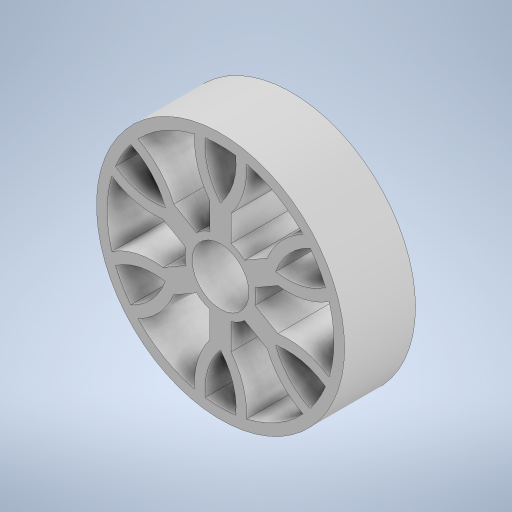
# Autodesk Inventor part: kumandaiç
Saved by Autodesk Inventor 2023 (Build 270158000, 158)
## iProperties
Created: 2023-01-31
Part Number: kumandaiç
Material: Generic
Document SubType Name: Modeling
Designer: Umut Yücesoy
Density: 1 g/cm^3
Appearance: Default
Author: Umut Yücesoy
Autodesk Inventor part; units mm, degrees
ref_plane "YZ Plane" through (0, 0, 0) normal (1, 0, 0) x (0, 1, 0)
ref_plane "XZ Plane" through (0, 0, 0) normal (0, 1, 0) x (-1, 0, 0)
ref_plane "XY Plane" through (0, 0, 0) normal (0, 0, 1) x (1, 0, 0)
sketch "Sketch1" plane through (0, 0, 0) normal (0, 0, 1) x (1, 0, 0)
  circle A0 centre (0, 0) radius 17.5
  circle A1 centre (0, 0) radius 5
  line L0 (0, 5) -> (0, 9)
  arc A2 (0, 9) -> (1.8691, 17.3999) centre (-7.0076, 14.9672) ccw
  arc A3 (1.5, 8.4713) -> (3.471, 17.1523) centre (-7.0076, 14.9672) ccw
  line L1 (1.5, 8.4713) -> (1.5, 4.7697)
  arc A4 (-1.8691, 17.3999) -> (0, 9) centre (7.0076, 14.9672) ccw
  arc A5 (-3.471, 17.1523) -> (-1.5, 8.4713) centre (7.0076, 14.9672) ccw
  line L2 (-1.5, 8.4713) -> (-1.5, 4.7697)
  arc A6 (-6.5864, 5.5347) -> (-13.1189, 11.5821) centre (-16.4658, 1.4148) ccw
  arc A7 (-7.7942, 4.5) -> (-14.1342, 10.3186) centre (-16.4658, 1.4148) ccw
  line L3 (-6.5864, 5.5347) -> (-3.3807, 3.6839)
  line L4 (-4.3301, 2.5) -> (-7.7942, 4.5)
  line L5 (-8.0864, 2.9366) -> (-4.8807, 1.0858)
  arc A8 (-16.5898, 5.5702) -> (-8.0864, 2.9366) centre (-9.4581, 13.5524) ccw
  arc A9 (-16.0033, 7.0813) -> (-7.7942, 4.5) centre (-9.4581, 13.5524) ccw
  arc A10 (-8.0864, -2.9366) -> (-16.5898, -5.5702) centre (-9.4581, -13.5524) ccw
  arc A11 (-7.7942, -4.5) -> (-16.0033, -7.0813) centre (-9.4581, -13.5524) ccw
  line L6 (-8.0864, -2.9366) -> (-4.8807, -1.0858)
  line L7 (-4.3301, -2.5) -> (-7.7942, -4.5)
  line L8 (-6.5864, -5.5347) -> (-3.3807, -3.6839)
  arc A12 (-13.1189, -11.5821) -> (-6.5864, -5.5347) centre (-16.4658, -1.4148) ccw
  arc A13 (-14.1342, -10.3186) -> (-7.7942, -4.5) centre (-16.4658, -1.4148) ccw
  arc A14 (-1.5, -8.4713) -> (-3.471, -17.1523) centre (7.0076, -14.9672) ccw
  arc A15 (0, -9) -> (-1.8691, -17.3999) centre (7.0076, -14.9672) ccw
  line L9 (-1.5, -8.4713) -> (-1.5, -4.7697)
  line L10 (0, -5) -> (0, -9)
  line L11 (1.5, -8.4713) -> (1.5, -4.7697)
  arc A16 (3.471, -17.1523) -> (1.5, -8.4713) centre (-7.0076, -14.9672) ccw
  arc A17 (1.8691, -17.3999) -> (0, -9) centre (-7.0076, -14.9672) ccw
  arc A18 (6.5864, -5.5347) -> (13.1189, -11.5821) centre (16.4658, -1.4148) ccw
  arc A19 (7.7942, -4.5) -> (14.1342, -10.3186) centre (16.4658, -1.4148) ccw
  line L12 (6.5864, -5.5347) -> (3.3807, -3.6839)
  line L13 (4.3301, -2.5) -> (7.7942, -4.5)
  line L14 (8.0864, -2.9366) -> (4.8807, -1.0858)
  arc A20 (16.5898, -5.5702) -> (8.0864, -2.9366) centre (9.4581, -13.5524) ccw
  arc A21 (16.0033, -7.0813) -> (7.7942, -4.5) centre (9.4581, -13.5524) ccw
  arc A22 (8.0864, 2.9366) -> (16.5898, 5.5702) centre (9.4581, 13.5524) ccw
  arc A23 (7.7942, 4.5) -> (16.0033, 7.0813) centre (9.4581, 13.5524) ccw
  line L15 (8.0864, 2.9366) -> (4.8807, 1.0858)
  line L16 (4.3301, 2.5) -> (7.7942, 4.5)
  line L17 (6.5864, 5.5347) -> (3.3807, 3.6839)
  arc A24 (13.1189, 11.5821) -> (6.5864, 5.5347) centre (16.4658, 1.4148) ccw
  arc A25 (14.1342, 10.3186) -> (7.7942, 4.5) centre (16.4658, 1.4148) ccw
  circle A26 centre (0, 0) radius 4
  circle A27 centre (0, 0) radius 16
  point P0 (2.1535, 15.8544)
  point P1 (-2.1535, 15.8544)
  point P2 (15.3247, -4.5992)
  point P3 (15.3247, 4.5992)
  point P4 (3.6793, 15.5712)
  point P5 (11.6454, 10.972)
  point P6 (14.8071, 6.0622)
  point P7 (12.6536, 9.7922)
  point P8 (14.8071, -6.0622)
  point P9 (12.6536, -9.7922)
  point P10 (2.1535, -15.8544)
  point P11 (-2.1535, -15.8544)
  point P12 (11.6454, -10.972)
  point P13 (3.6793, -15.5712)
  point P14 (-3.6793, -15.5712)
  point P15 (-11.6454, -10.972)
  point P16 (-12.6536, -9.7922)
  point P17 (-14.8071, -6.0622)
  point P18 (-15.3247, -4.5992)
  point P19 (-15.3247, 4.5992)
  point P20 (-3.6793, 15.5712)
  point P21 (-11.6454, 10.972)
  point P22 (-14.8071, 6.0622)
  point P23 (-12.6536, 9.7922)
  dimension "d10" = 32
  dimension "d0" = 35
  dimension "d1" = 10
  dimension "d2" = 4
  dimension "d3" = 1.5
  dimension "d4" = 0
  dimension "d7" = 360
  dimension "d9" = 8
  constraints: 52 point on circle, 36 end point, 27 centre point, 5 symmetric about line, 4 coincident, 1 vertical, 119 other
  measures "d0" diameter of A0
  measures "d1" diameter of A1
  measures "d2" distance of L0.start L0.end
  measures "d3" radial gap between concentric circles of A2 A3
  measures "d4" distance from line of point (0, 0) L0
  measures "d9" diameter of A26
extrude "Extrusion1" add sketch "Sketch1" against normal blind 10 contours A0 A20 A27 A22 | A22 A27 A23 A0 | A0 A21 A27 A20 | A23 A27 A25 A0 | A22 L15 A1 L16 A23 A27 | A0 A19 A27 A21 | A27 A21 L13 A1 L14 A20 | A25 A27 A24 A0 | A0 A18 A27 A19 | A24 A27 A3 A0 | A25 L16 A1 L17 A24 A27 | A1 | A0 A16 A27 A18 | A27 A18 L12 A1 L13 A19 | A3 A27 A2 A0 | A0 A17 A27 A16 | A2 A27 A4 A0 | A3 L1 A1 L0 A2 A27 | A0 A15 A27 A17 | A27 A17 L10 A1 L11 A16 | A4 A27 A5 A0 | A0 A14 A27 A15 | A5 A27 A6 A0 | A4 L0 A1 L2 A5 A27 | A0 A12 A27 A14 | A27 A14 L9 A1 L10 A15 | A6 A27 A7 A0 | A0 A13 A27 A12 | A7 A27 A9 A0 | A6 L3 A1 L4 A7 A27 | A0 A11 A27 A13 | A27 A13 L7 A1 L8 A12 | A9 A27 A8 A0 | A1 L5 A8 A27 A9 L4 | A0 A10 A27 A11 | L7 A11 A27 A10 L6 A1 | A8 A27 A10 A0
body "Solid1"
